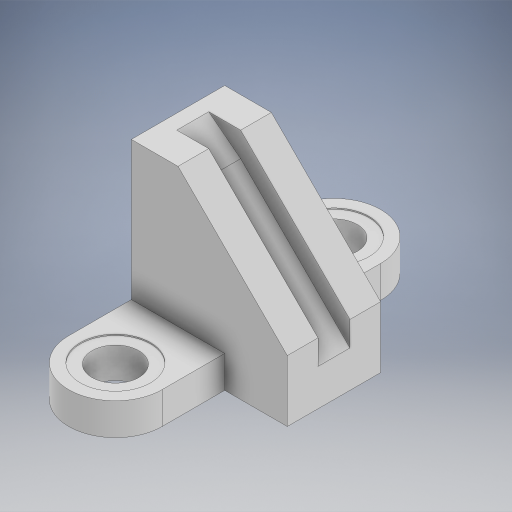
# Autodesk Inventor part: LE-1.3
Saved by Autodesk Inventor 2024 (Build 280153000, 153)
## iProperties
Created: 2024-01-25
Part Number: LE-1.3
Material: Generic
Document SubType Name: Modeling
Designer: Alex
Density: 1 g/cm^3
Appearance: Default
Author: Alex
Autodesk Inventor part; units mm, degrees
ref_plane "YZ Plane" through (0, 0, 0) normal (1, 0, 0) x (0, 1, 0)
sketch "Sketch1" plane through (0, 0, 0) normal (0, 1, 0) x (-1, 0, 0)
  arc A0 (76, -38) -> (0, -38) centre (38, -38) ccw
  line L0 (101.4, 0) -> (-76.4, 0) projected
  line L1 (0, -304.8) -> (0, 50.8) projected
  line L2 (76, -38) -> (76, -216)
  line L3 (0, -38) -> (0, -216)
  line L4 (76, -216) -> (0, -216) construction
  arc A1 (0, -216) -> (76, -216) centre (38, -216) ccw
  circle A2 centre (38, -38) radius 28.5
  circle A3 centre (38, -38) radius 19
  circle A4 centre (38, -216) radius 28.5
  circle A5 centre (38, -216) radius 19
  line L5 (76, -127) -> (0, -127) construction
  line L6 (0, -89) -> (76, -89) construction
  line L7 (76, -89) -> (76, -165) construction
  line L8 (76, -165) -> (0, -165) construction
  line L9 (0, -165) -> (0, -89) construction
  line L10 (0, -89) -> (76, -165) construction
  line L11 (76, -89) -> (0, -165) construction
  line L12 (76, -89) -> (-51, -89)
  line L13 (-51, -89) -> (-51, -165)
  line L14 (-51, -165) -> (76, -165)
  line L15 (76, -165) -> (76, -89)
  point P0 (0, 0)
  point P1 (38, -127)
  point P2 (0, -165)
  point P3 (0, -89)
  dimension "d0" = 76
  dimension "d1" = 178
  dimension "d3" = 57
  dimension "d4" = 38
  dimension "d5" = 57
  dimension "d6" = 38
  dimension "d7" = 76
  dimension "d8" = 127
  dimension "d9" = 165
  constraints: 28 end point, 6 centre point, 6 midpoint, 4 coincident, 4 parallel, 4 point on circle, 4 tangent, 3 horizontal, 3 point on line, 2 perpendicular, 1 vertical
  measures "d0" diameter of A0
  measures "d1" distance of L2.start L2.end
  measures "d3" diameter of A2
  measures "d4" diameter of A3
  measures "d5" diameter of A4
  measures "d6" diameter of A5
  measures "d7" distance of L6.end L7.end
  measures "d8" distance of L14.end L13.end
  measures "d9" distance between parallel lines of L14 L0
extrude "Extrusion1" add sketch "Sketch1" along normal blind 26 contours L2 L12 L1 A0 | L2 A1 L1 L14 | A2 | A3 | A4 | A5
sketch "Sketch2" plane through (0, 26, 0) normal (0, 1, 0) x (1, 0, 0)
  line L0 (-76, 165) -> (0, 165) projected
  line L1 (-76, 165) -> (0, 165) projected
  line L2 (-76, 165) -> (0, 165) projected
  line L3 (-76, 165) -> (0, 165) projected
  line L4 (0, 165) -> (0, 216) projected
  line L5 (0, 165) -> (0, 216) projected
  line L6 (-76, 216) -> (-76, 165) projected
  line L7 (0, 165) -> (0, 216) projected
  line L8 (0, 165) -> (0, 216) projected
  line L9 (-76, 216) -> (-76, 165) projected
  line L10 (-76, 216) -> (-76, 165) projected
  arc A0 (0, 216) -> (-76, 216) centre (-38, 216) ccw projected
  line L11 (0, 165) -> (0, 216) projected
  arc A1 (0, 216) -> (-76, 216) centre (-38, 216) ccw projected
  line L12 (-76, 216) -> (-76, 165) projected
  line L13 (-76, 165) -> (0, 165) projected
  arc A2 (0, 216) -> (-76, 216) centre (-38, 216) ccw projected
  arc A3 (0, 216) -> (-76, 216) centre (-38, 216) ccw projected
  arc A4 (0, 216) -> (-76, 216) centre (-38, 216) ccw projected
  line L14 (0, 165) -> (0, 216) projected
  line L15 (-76, 165) -> (0, 165) projected
  line L16 (-76, 216) -> (-76, 165) projected
  arc A5 (0, 216) -> (-76, 216) centre (-38, 216) ccw projected
  line L17 (-76, 216) -> (-76, 165) projected
  line L18 (-76, 89) -> (-76, 38) projected
  line L19 (-76, 89) -> (-76, 38) projected
  line L20 (0, 89) -> (-76, 89) projected
  line L21 (0, 89) -> (-76, 89) projected
  line L22 (0, 89) -> (-76, 89) projected
  line L23 (0, 89) -> (-76, 89) projected
  line L24 (0, 38) -> (0, 89) projected
  line L25 (0, 38) -> (0, 89) projected
  line L26 (-76, 89) -> (-76, 38) projected
  line L27 (-76, 89) -> (-76, 38) projected
  line L28 (0, 38) -> (0, 89) projected
  line L29 (0, 38) -> (0, 89) projected
  line L30 (-76, 89) -> (-76, 38) projected
  line L31 (0, 89) -> (-76, 89) projected
  line L32 (0, 38) -> (0, 89) projected
  arc A6 (-76, 38) -> (0, 38) centre (-38, 38) ccw projected
  line L33 (-76, 89) -> (-76, 38) projected
  arc A7 (-76, 38) -> (0, 38) centre (-38, 38) ccw projected
  line L34 (0, 38) -> (0, 89) projected
  line L35 (0, 89) -> (-76, 89) projected
  arc A8 (-76, 38) -> (0, 38) centre (-38, 38) ccw projected
  arc A9 (-76, 38) -> (0, 38) centre (-38, 38) ccw projected
  arc A10 (-76, 38) -> (0, 38) centre (-38, 38) ccw projected
  arc A11 (-76, 38) -> (0, 38) centre (-38, 38) ccw projected
  circle A12 centre (-38, 38) radius 19 projected
  circle A13 centre (-38, 38) radius 28.5 projected
  line L36 (-101.4, 0) -> (76.4, 0) projected
  arc A14 (-76, 38) -> (0, 38) centre (-38, 38) ccw projected
  line L37 (-76, 165) -> (0, 165) construction
  line L38 (-76, 216) -> (0, 216) construction
  circle A15 centre (-38, 216) radius 19 projected
  circle A16 centre (-38, 216) radius 28.5 projected
  arc A17 (0, 216) -> (-76, 216) centre (-38, 216) ccw projected
  line L39 (-76, 89) -> (51, 89) projected
  line L40 (0, 89) -> (-76, 89) construction
  line L41 (-76, 127) -> (0, 127) construction
  line L42 (-76, 89) -> (-76, 165) construction
  line L43 (0, 165) -> (0, 89) construction
  line L44 (0, 89) -> (-76, 165) construction
  line L45 (-76, 89) -> (0, 165) construction
  line L46 (-76, 165) -> (-76, 89) projected
  line L47 (51, 89) -> (51, 165) projected
  line L48 (-76, 38) -> (-76, 216) projected
  line L49 (0, 38) -> (0, 216) projected
  line L50 (51, 165) -> (-76, 165) projected
  point P0 (0, 0)
  point P1 (0, 0)
  point P2 (-38, 127)
  constraints: 18 other
extrude "Extrusion2" cut sketch "Sketch2" against normal blind 1 contours A13 | A16
extrude "Extrusion3" cut sketch "Sketch2" against normal up to surface (26 mm away) contours A12 | A15
extrude "Extrusion4" add sketch "Sketch1" along normal blind 50 contours L2 L14 L1 L12 | L1 L14 L13 L12
sketch "Sketch3" plane through (0, 0, -89) normal (0, 0, 1) x (1, 0, 0)
  line L0 (51, 50) -> (-76, 50) construction
  line L1 (-76, 26) -> (-76, 50) construction
  line L2 (-76, 0) -> (-76, 26) construction
  line L3 (0, 0) -> (-76, 0) construction
  line L4 (51, 0) -> (0, 0) construction
  line L5 (51, 0) -> (51, 50) construction
  line L6 (51, 50) -> (-38, 139)
  line L7 (51, 50) -> (230.6051, 50) construction
  line L8 (-76, 139) -> (-76, 50)
  line L9 (-76, 139) -> (-38, 139)
  line L10 (-76, 50) -> (51, 50)
  dimension "d18" = 135
  dimension "d19" = 38
  constraints: 10 end point, 2 collinear, 2 horizontal
  measures "d18" angle of L7 L6
  measures "d19" distance of L6.end L8.start
extrude "Extrusion5" add sketch "Sketch3" against normal up to surface (76 mm away)
ref_plane "Work Plane1" through (-38, 139, -89) normal (0.7071068, -0.7071068, 0) x (0, 0, -1)
sketch "Sketch4" plane through (-76, 139, -89) normal (0, 1, 0) x (1, 0, 0)
  line L0 (38, 76) -> (0, 76) construction
  line L1 (0, 0) -> (0, 76) construction
  line L2 (38, 0) -> (0, 0) construction
  line L3 (38, 0) -> (38, 76) construction
  line L4 (38, 38) -> (38, 25) construction
  line L5 (38, 25) -> (12, 25)
  line L6 (12, 25) -> (12, 51)
  line L7 (12, 51) -> (38, 51)
  line L8 (38, 51) -> (38, 25)
  point P0 (76, -89)
  dimension "d23" = 13
  dimension "d24" = 26
  dimension "d25" = 26
  constraints: 10 end point, 2 parallel, 1 horizontal, 1 midpoint, 1 perpendicular, 1 point on line
  measures "d23" distance of L4.start L4.end
  measures "d24" distance of L6.end L7.end
  measures "d25" distance of L5.end L6.end
ref_plane "Work Plane2" through (-64, 139, -114) normal (-0.6120345, -0.7908311, 0) x (0, 0, -1)
extrude "Extrusion6" cut sketch "Sketch4" along normal up to surface surface through (-64, 139, -114) normal (-0.6120345, -0.7908311, 0)
sketch "Sketch5" plane through (-38, 139, -89) normal (0.7071068, -0.7071068, 0) x (0, 0, -1)
  line L0 (25, -14.2282) -> (51, -14.2282) projected
  line L1 (25, 0) -> (25, -14.2282) projected
  line L2 (25, 0) -> (51, 0) projected
  line L3 (51, 0) -> (51, -14.2282) projected
  point P0 (-89, -71.4178)
extrude "Extrusion7" cut sketch "Sketch5" along normal up to surface surface through (51, 0, -89) normal (1, 0, 0)
body "Solid1"
